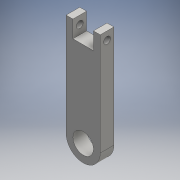
# Autodesk Inventor part: promo2
Saved by Autodesk Inventor 2016 (Build 200138000, 138)
## iProperties
Created: 2016-05-06
Part Number: promo2
Material: 一般
Document SubType Name: Modeling
Designer: 宏太
Density: 1 g/cm^3
Appearance: 既定
Author: 宏太
Autodesk Inventor part; units mm, degrees
ref_plane "YZ Plane" through (0, 0, 0) normal (1, 0, 0) x (0, 1, 0)
ref_plane "XZ Plane" through (0, 0, 0) normal (0, 1, 0) x (-1, 0, 0)
ref_plane "XY Plane" through (0, 0, 0) normal (0, 0, 1) x (1, 0, 0)
sketch "スケッチ1" plane through (0, 0, 0) normal (0, 1, 0) x (-1, 0, 0)
  line L0 (-5, 17.5) -> (5, -17.5) construction
  line L1 (5, 17.5) -> (-5, -17.5) construction
  arc A0 (-5, -12.5) -> (5, -12.5) centre (0, -12.5) ccw
  line L2 (5, 17.5) -> (-5, 17.5)
  line L3 (5, 17.5) -> (5, -12.5)
  line L4 (-5, 17.5) -> (-5, -12.5)
  point P0 (0, 0)
  dimension "d0" = 10
  dimension "d1" = 35
  constraints: 10 end point, 2 midpoint, 2 point on circle, 2 vertical, 1 centre point, 1 horizontal, 1 tangent
  measures "d0" distance of L0.end L1.end
  measures "d1" distance of L1.start L0.end
extrude "押し出し1" add sketch "スケッチ1" along normal blind 4
sketch "スケッチ2" plane through (0, 0, 0) normal (0, 1, 0) x (-1, 0, 0)
  arc A0 (-5, -12.5) -> (5, -12.5) centre (0, -12.5) ccw projected
  circle A1 centre (0, -12.5) radius 3
  point P0 (0, 0)
  dimension "d7" = 6
  constraints: 1 centre point, 1 coincident
  measures "d7" diameter of A1
extrude "押し出し2" cut sketch "スケッチ2" along normal blind 4
sketch "スケッチ3" plane through (0, 0, 0) normal (0, 1, 0) x (-1, 0, 0)
  line L0 (-5, 17.5) -> (5, 17.5) projected
  line L1 (3, 17.5) -> (3, 12.5)
  line L2 (3, 17.5) -> (8, 17.5) construction
  line L3 (3, 12.5) -> (-3, 12.5)
  line L4 (3, 12.5) -> (9, 12.5) construction
  line L5 (-3, 12.5) -> (-3, 17.5)
  line L6 (-3, 17.5) -> (3, 17.5)
  point P0 (0, 0)
  dimension "d10" = 5
  dimension "d11" = 270
  dimension "d12" = 6
  dimension "d13" = 180
  constraints: 12 end point, 3 horizontal, 2 equal length, 2 perpendicular, 2 point on line, 1 collinear
  measures "d10" distance of L1.start L1.end
  measures "d12" distance of L1.end L3.end
  measures "d13" angle of L3 L4
extrude "押し出し3" cut sketch "スケッチ3" along normal blind 4
sketch "スケッチ4" plane through (0, 0, 0) normal (1, 0, 0) x (0, 1, 0)
  circle A0 centre (2, 15.1228) radius 1
  line L0 (0, -12.5) -> (0, 17.5) projected
  point P0 (0, 0)
  dimension "d16" = 2
  dimension "d18" = 2
  constraints: 1 centre point
  measures "d16" diameter of A0
  measures "d18" distance from line of L0 A0.centre
extrude "押し出し4" cut sketch "スケッチ4" along normal mid plane 10
